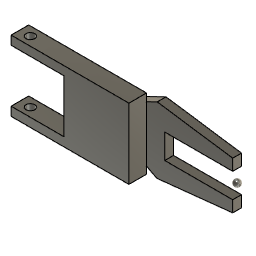
RollArm (stilizzato) Fusion360 (Autodesk Fusion 360 archive; units mm, degrees)
design "rollarm asse 3"
Autodesk Fusion 360 part; units mm, degrees
sketch "Schizzo1" plane through (0, 0, 0) normal (0, 0, 1) x (1, 0, 0)
  line L0 (-70, 25) -> (-3, 25)
  line L1 (-3, 25) -> (-3, 15)
  line L2 (-3, 15) -> (-70, 15)
  line L3 (-70, 15) -> (-70, 25)
  circle A0 centre (-64, 20) radius 2.5
  line L4 (-70, 20) -> (-64, 20) construction
  dimension "d1" = 67
  dimension "d2" = 10
  dimension "d3" = 5
  dimension "d12" = 6
  constraint horizontal L0
  constraint vertical L1
  constraint horizontal L2
  constraint vertical L3
  constraint midpoint L3 L4.start
  constraint coincident A0.centre L4.end
  measures "d1" distance of L0.start L0.end
  measures "d2" distance of L0.start L2.end
  measures "d3" diameter of A0
  measures "d12" distance of L4.start A0.centre
extrude "Estrusione1" add sketch "Schizzo1" along normal blind 40 makes body 1
sketch "Schizzo2" plane through (0, 15, 0) normal (0, -1, 0) x (1, 0, 0)
  line L0 (-70, 0) -> (-3, 0)
  line L1 (-3, 0) -> (-3, 40)
  line L2 (-3, 40) -> (-70, 40)
  line L3 (-70, 40) -> (-70, 0)
  line L4 (-70, 35) -> (-40, 35)
  line L5 (-40, 35) -> (-40, 5)
  line L6 (-40, 5) -> (-70, 5)
  line L7 (-70, 5) -> (-70, 35)
  dimension "d6" = 5
  dimension "d7" = 5
  dimension "d8" = 30
  constraint horizontal L4
  constraint vertical L5
  constraint horizontal L6
  constraint vertical L7
  constraint collinear L3 L7
  measures "d6" distance of L2 L4
  measures "d7" distance of L0 L6
  measures "d8" distance of L3 L5
extrude "Estrusione2" cut sketch "Schizzo2" against normal through all contours L3 L4 L5 L6 L7 bodies 1
sketch "Schizzo3" plane through (0, 25, 0) normal (0, 1, 0) x (-1, 0, 0)
  line L0 (40, 35) -> (70, 35)
  line L1 (70, 35) -> (70, 40)
  line L2 (70, 40) -> (3, 40)
  line L3 (3, 40) -> (3, 0)
  line L4 (3, 0) -> (70, 0)
  line L5 (70, 0) -> (70, 5)
  line L6 (70, 5) -> (40, 5)
  line L7 (40, 5) -> (40, 35)
  line L8 (12.3168, 8.8043) -> (12.3168, 31.1957)
  line L9 (12.3168, 31.1957) -> (-3.0953, 38.6446)
  line L10 (-3.0953, 38.6446) -> (-46, 32.4046)
  line L11 (-46, 32.4046) -> (-46, 25.947)
  line L12 (-46, 25.947) -> (-7.3656, 25.947)
  line L13 (-7.3656, 25.947) -> (-7.3656, 11.9386)
  line L14 (-7.3656, 11.9386) -> (-46, 11.9386)
  line L15 (-46, 11.9386) -> (-46, 5.481)
  line L16 (-46, 5.481) -> (-2.8832, 0.9317)
  line L17 (-2.8832, 0.9317) -> (12.3168, 8.8043)
  line L18 (12.3168, 20) -> (3, 20)
  dimension "d13" = 116
  constraint perpendicular L4 L8
  constraint parallel L3 L11
  constraint perpendicular L11 L12
  constraint perpendicular L12 L13
  constraint perpendicular L13 L14
  constraint perpendicular L14 L15
  constraint equal L9 L17
  constraint equal L10 L16
  constraint equal L11 L15
  constraint equal L12 L14
  constraint midpoint L8 L18.start
  constraint perpendicular L8 L18
  constraint midpoint L3 L18.end
  measures "d13" distance of L1 L11
extrude "Estrusione3" add sketch "Schizzo3" along normal blind 5 separate body contours L3 L8 L9 L18 | L3 L9 L10 L11 L12 L13 L14 L15 L16 L17 | L3 L8 L17 L18 makes body 2
ref_plane "Piano di lavoro1" through (26.6828, 27.5, 18.9428) normal (0, 0, 1) x (1, 0, 0)
sketch "Schizzo4" plane through (26.6828, 27.5, 18.9428) normal (0, 0, 1) x (1, 0, 0)
  line L0 (19.3179, 1.9508) -> (19.3179, -1.9508)
  arc A0 (19.3179, -1.9508) -> (19.3179, 1.9508) centre (19.3172, 0) ccw
  line L1 (19.3172, -2.5) -> (19.3172, 2.5)
  constraint vertical L0
  constraint midpoint A0.centre L1
revolve "Rivoluzione1" add sketch "Schizzo4" angle 360 about axis through (46.0007, 29.4508, 18.9428) along (0, -1, 0) separate body makes body 3
equation "d13 = 110 mm + 6 mm"

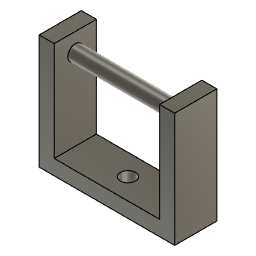
design "rollarm asse 1"
Autodesk Fusion 360 part; units mm, degrees
sketch "Schizzo1" plane through (0, 0, 0) normal (0, 0, 1) x (1, 0, 0)
  line L0 (-26.2044, 17.7042) -> (18.7956, 17.7042)
  line L1 (18.7956, 17.7042) -> (18.7956, 3.7042)
  line L2 (18.7956, 3.7042) -> (-26.2044, 3.7042)
  line L3 (-26.2044, 3.7042) -> (-26.2044, 17.7042)
  line L4 (-3.7044, 17.7042) -> (-3.7044, 3.7042) construction
  circle A0 centre (-3.7044, 10.7042) radius 2.5
  dimension "d1" = 14
  dimension "d2" = 45
  dimension "d3" = 5
  constraint horizontal L0
  constraint vertical L1
  constraint horizontal L2
  constraint vertical L3
  constraint midpoint L0 L4.start
  constraint midpoint L2 L4.end
  constraint midpoint L4 A0.centre
  measures "d1" distance of L0.start L2.end
  measures "d2" distance of L0.start L0.end
  measures "d3" diameter of A0
extrude "Estrusione1" add sketch "Schizzo1" along normal blind 5
sketch "Schizzo2" plane through (0, 0, 5) normal (0, 0, 1) x (-1, 0, 0)
  circle A0 centre (3.7044, -10.7042) radius 2.5
  line L0 (26.2044, -3.7042) -> (-18.7956, -3.7042)
  line L1 (-18.7956, -3.7042) -> (-18.7956, -17.7042)
  line L2 (-18.7956, -17.7042) -> (26.2044, -17.7042)
  line L3 (26.2044, -17.7042) -> (26.2044, -3.7042)
  line L4 (-18.7956, -3.7042) -> (-13.7956, -3.7042)
  line L5 (-13.7956, -3.7042) -> (-13.7956, -17.7042)
  line L6 (-13.7956, -17.7042) -> (-18.7956, -17.7042)
  line L7 (-18.7956, -17.7042) -> (-18.7956, -3.7042)
  line L8 (21.2044, -3.7042) -> (26.2044, -3.7042)
  line L9 (26.2044, -3.7042) -> (26.2044, -17.7042)
  line L10 (26.2044, -17.7042) -> (21.2044, -17.7042)
  line L11 (21.2044, -17.7042) -> (21.2044, -3.7042)
  dimension "d6" = 5
  constraint horizontal L4
  constraint vertical L5
  constraint horizontal L6
  constraint vertical L7
  constraint horizontal L8
  constraint vertical L9
  constraint horizontal L10
  constraint vertical L11
  constraint collinear L0 L8
  constraint collinear L0 L4
  constraint collinear L1 L7
  constraint collinear L2 L6
  constraint collinear L2 L10
  constraint collinear L3 L9
  constraint equal L4 L8
  measures "d6" distance of L0.end L4.end
extrude "Estrusione2" add sketch "Schizzo2" along normal blind 33 contours L0 L2 L3 L8 L9 L10 L11 | L0 L1 L2 L4 L5 L6 L7
sketch "Schizzo3" plane through (18.7956, 0, 0) normal (1, 0, 0) x (0, 1, 0)
  line L0 (3.7042, 0) -> (17.7042, 0)
  line L1 (17.7042, 0) -> (17.7042, 38)
  line L2 (17.7042, 38) -> (3.7042, 38)
  line L3 (3.7042, 38) -> (3.7042, 0)
  circle A0 centre (10.7042, 32) radius 2.5
  line L4 (10.7042, 38) -> (10.7042, 32)
  dimension "d9" = 5
  dimension "d10" = 6
  constraint midpoint L2 L4.start
  constraint perpendicular L2 L4
  constraint coincident A0.centre L4.end
  measures "d9" diameter of A0
  measures "d10" distance of L4.start A0.centre
extrude "Estrusione3" add sketch "Schizzo3" against normal up to surface (40 mm away) contours A0
equation "d7 = 32 mm - 5 mm + 6 mm"

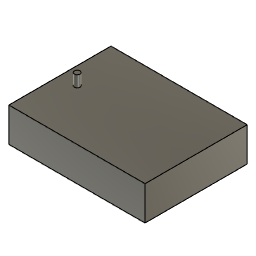
design "base rollarm"
Autodesk Fusion 360 part; units mm, degrees
sketch "Schizzo1" plane through (0, 0, 0) normal (0, 0, 1) x (1, 0, 0)
  line L0 (-90, 40) -> (30, 40)
  line L1 (30, 40) -> (30, -50)
  line L2 (30, -50) -> (-90, -50)
  line L3 (-90, -50) -> (-90, 40)
  dimension "d1" = 90
  dimension "d2" = 120
  constraint horizontal L0
  constraint vertical L1
  constraint horizontal L2
  constraint vertical L3
  measures "d1" distance of L0.start L2.end
  measures "d2" distance of L0.start L0.end
extrude "Estrusione1" add sketch "Schizzo1" along normal blind 30
sketch "Schizzo2" plane through (0, 0, 30) normal (0, 0, 1) x (-1, 0, 0)
  line L0 (90, 50) -> (-30, 50)
  line L1 (-30, 50) -> (-30, -40)
  line L2 (-30, -40) -> (90, -40)
  line L3 (90, -40) -> (90, 50)
  circle A0 centre (74.7461, 5) radius 2.5
  line L4 (74.7461, 5) -> (90, 5) construction
  dimension "d5" = 5
  constraint coincident A0.centre L4.start
  constraint coincident L3 L4.end
  constraint perpendicular L3 L4
  constraint midpoint L3 L4.end
  measures "d5" diameter of A0
extrude "Estrusione2" add sketch "Schizzo2" along normal blind 10 contours A0

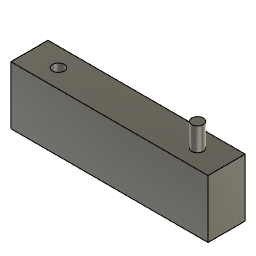
design "rollarm asse 2"
Autodesk Fusion 360 part; units mm, degrees
sketch "Schizzo1" plane through (0, 0, 0) normal (0, 0, 1) x (1, 0, 0)
  line L0 (-90, 25) -> (-5, 25)
  line L1 (-5, 25) -> (-5, 9)
  line L2 (-5, 9) -> (-90, 9)
  line L3 (-90, 9) -> (-90, 25)
  line L4 (-90, 17) -> (-77.5, 17) construction
  circle A0 centre (-77.5, 17) radius 2.5
  dimension "d1" = 85
  dimension "d2" = 16
  dimension "d3" = 12.5
  dimension "d4" = 5
  constraint horizontal L0
  constraint vertical L1
  constraint horizontal L2
  constraint vertical L3
  constraint midpoint L3 L4.start
  constraint perpendicular L3 L4
  constraint coincident L4.end A0.centre
  measures "d1" distance of L0.start L0.end
  measures "d2" distance of L0.start L2.end
  measures "d3" distance of L4.start L4.end
  measures "d4" diameter of A0
extrude "Estrusione1" add sketch "Schizzo1" along normal blind 25
sketch "Schizzo2" plane through (0, 0, 25) normal (0, 0, 1) x (-1, 0, 0)
  circle A0 centre (77.5, -17) radius 2.5
  line L0 (90, -9) -> (5, -9)
  line L1 (5, -9) -> (5, -25)
  line L2 (5, -25) -> (90, -25)
  line L3 (90, -25) -> (90, -9)
  circle A1 centre (17.5, -17) radius 2.5
  line L4 (77.5, -17) -> (17.5, -17) construction
  dimension "d7" = 5
  dimension "d8" = 60
  constraint coincident A0.centre L4.start
  constraint coincident A1.centre L4.end
  constraint parallel L2 L4
  measures "d7" diameter of A1
  measures "d8" distance of A0.centre A1.centre
extrude "Estrusione2" add sketch "Schizzo2" along normal blind 10 contours A1
